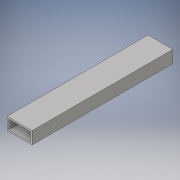
# Autodesk Inventor part: Cross 2 x 1 beam on bottom of elevator
Saved by Autodesk Inventor 2016 SP2 (Build 200236200, 236)
## iProperties
Created: 2018-01-27
Part Number: Cross 2 x 1 beam on bottom of elevator
Material: Generic
Document SubType Name: Modeling
Designer: CAD
Density: 1 g/cm^3
Appearance: Default
Author: CAD
Autodesk Inventor part; units mm, degrees
ref_plane "YZ Plane" through (0, 0, 0) normal (1, 0, 0) x (0, 1, 0)
ref_plane "XZ Plane" through (0, 0, 0) normal (0, 1, 0) x (-1, 0, 0)
ref_plane "XY Plane" through (0, 0, 0) normal (0, 0, 1) x (1, 0, 0)
sketch "Sketch1" plane through (0, 0, 0) normal (0, 0, 1) x (1, 0, 0)
  line L0 (0, 0) -> (0, 25.4)
  line L1 (0, 25.4) -> (50.8, 25.4)
  line L2 (50.8, 25.4) -> (50.8, 0)
  line L3 (50.8, 0) -> (0, 0)
  line L4 (3.175, 3.175) -> (3.175, 22.225)
  line L5 (3.175, 22.225) -> (47.625, 22.225)
  line L6 (47.625, 22.225) -> (47.625, 3.175)
  line L7 (47.625, 3.175) -> (3.175, 3.175)
  dimension "d0" = 25.4
  dimension "d1" = 50.8
  dimension "d2" = 3.175
  constraints: 16 end point, 6 perpendicular, 1 vertical, 3 other
  measures "d0" distance of L0.start L0.end
  measures "d1" distance of L0.end L1.end
  measures "d2" distance between parallel lines of L3 L7
extrude "Extrusion1" add sketch "Sketch1" along normal blind 287.3375
body "Solid1"
